Autodesk Fusion 360 part; units mm, degrees
(part 11 of 11)
  spline S89 degree 5 poles (-2.0699, -13.4086) (-2.0698, -13.4117) (-2.0696, -13.4179) (-2.0693, -13.4271) (-2.0688, -13.4395) (-2.0682, -13.4548) (-2.0675, -13.4702) (-2.0667, -13.4855) (-2.0659, -13.5008) (-2.065, -13.516) (-2.064, -13.5312) (-2.063, -13.5464) (-2.0619, -13.5616) (-2.0607, -13.5768) (-2.0595, -13.5919) (-2.0582, -13.6069) (-2.0568, -13.622) (-2.0553, -13.637) (-2.0538, -13.652) (-2.0522, -13.667) (-2.0506, -13.6819) (-2.0488, -13.6968) (-2.047, -13.7116) (-2.0452, -13.7265) (-2.0432, -13.7412) (-2.0412, -13.756) (-2.0391, -13.7707) (-2.0369, -13.7854) (-2.0347, -13.8) (-2.0324, -13.8147) (-2.03, -13.8292) (-2.0275, -13.8438) (-2.025, -13.8583) (-2.0224, -13.8727) (-2.0197, -13.8872) (-2.0169, -13.9015) (-2.0141, -13.9159) (-2.0112, -13.9302) (-2.0082, -13.9444) (-2.0051, -13.9587) (-2.0019, -13.9728) (-1.9987, -13.987) (-1.9954, -14.001) (-1.992, -14.0151) (-1.9885, -14.0291) (-1.9849, -14.043) (-1.9812, -14.0569) (-1.9775, -14.0708) (-1.9737, -14.0846) (-1.9697, -14.0983) (-1.9657, -14.112) (-1.9616, -14.1256) (-1.9574, -14.1392) (-1.9531, -14.1527) (-1.9487, -14.1662) (-1.9442, -14.1796) (-1.9396, -14.193) (-1.9349, -14.2063) (-1.9301, -14.2195) (-1.9252, -14.2327) (-1.9202, -14.2458) (-1.915, -14.2588) (-1.9097, -14.2717) (-1.9042, -14.2845) (-1.8986, -14.2972) (-1.8929, -14.3098) (-1.8871, -14.3224) (-1.8812, -14.335) (-1.8753, -14.3475) (-1.8691, -14.3598) (-1.8626, -14.3719) (-1.857, -14.3814) (-1.8526, -14.3883) (-1.8495, -14.3929) (-1.848, -14.3952) knots -1 -1 -1 -1 -1 -1 -0.98571429 -0.97142857 -0.95714286 -0.94285714 -0.92857143 -0.91428571 -0.9 -0.88571429 -0.87142857 -0.85714286 -0.84285714 -0.82857143 -0.81428571 -0.8 -0.78571429 -0.77142857 -0.75714286 -0.74285714 -0.72857143 -0.71428571 -0.7 -0.68571429 -0.67142857 -0.65714286 -0.64285714 -0.62857143 -0.61428571 -0.6 -0.58571429 -0.57142857 -0.55714286 -0.54285714 -0.52857143 -0.51428571 -0.5 -0.48571429 -0.47142857 -0.45714286 -0.44285714 -0.42857143 -0.41428571 -0.4 -0.38571429 -0.37142857 -0.35714286 -0.34285714 -0.32857143 -0.31428571 -0.3 -0.28571429 -0.27142857 -0.25714286 -0.24285714 -0.22857143 -0.21428571 -0.2 -0.18571429 -0.17142857 -0.15714286 -0.14285714 -0.12857143 -0.11428571 -0.1 -0.08571429 -0.07142857 -0.05714286 -0.04285714 -0.02857143 -0.01428571 0 0 0 0 0 0
  line L97 (-1.848, -14.3952) -> (-1.8092, -14.4516)
  arc A187 (-1.8651, -14.7929) -> (-1.8092, -14.4516) centre (-2.0153, -14.5931) ccw
  arc A188 (-1.8651, -14.7929) -> (-1.9565, -14.8631) centre (1.6741, -19.5) ccw
  arc A189 (-2.3006, -14.8287) -> (-1.9565, -14.8631) centre (-2.1106, -14.6662) ccw
  line L98 (-2.3006, -14.8287) -> (-2.3452, -14.7767)
  spline S90 degree 5 poles (-2.3452, -14.7767) (-2.3469, -14.7746) (-2.3506, -14.7705) (-2.3561, -14.7644) (-2.3639, -14.7566) (-2.3739, -14.7471) (-2.3842, -14.738) (-2.3947, -14.729) (-2.4053, -14.7201) (-2.416, -14.7112) (-2.4267, -14.7024) (-2.4375, -14.6937) (-2.4485, -14.6851) (-2.4596, -14.6766) (-2.4708, -14.6682) (-2.4821, -14.66) (-2.4936, -14.6519) (-2.5051, -14.6438) (-2.5168, -14.6359) (-2.5285, -14.628) (-2.5403, -14.6201) (-2.5521, -14.6124) (-2.5641, -14.6047) (-2.5761, -14.5971) (-2.5882, -14.5896) (-2.6004, -14.5822) (-2.6127, -14.5749) (-2.625, -14.5676) (-2.6374, -14.5604) (-2.6499, -14.5533) (-2.6624, -14.5462) (-2.675, -14.5392) (-2.6877, -14.5323) (-2.7005, -14.5254) (-2.7133, -14.5186) (-2.7261, -14.5119) (-2.7391, -14.5053) (-2.7521, -14.4987) (-2.7651, -14.4922) (-2.7782, -14.4857) (-2.7914, -14.4793) (-2.8047, -14.473) (-2.8179, -14.4667) (-2.8313, -14.4605) (-2.8447, -14.4544) (-2.8582, -14.4483) (-2.8717, -14.4423) (-2.8852, -14.4363) (-2.8989, -14.4304) (-2.9125, -14.4246) (-2.9263, -14.4188) (-2.9401, -14.4131) (-2.9539, -14.4075) (-2.9678, -14.4019) (-2.9817, -14.3964) (-2.9957, -14.3909) (-3.0097, -14.3855) (-3.0238, -14.3802) (-3.0379, -14.3749) (-3.0521, -14.3696) (-3.0663, -14.3645) (-3.0806, -14.3594) (-3.0949, -14.3543) (-3.1093, -14.3493) (-3.1237, -14.3444) (-3.1382, -14.3395) (-3.1527, -14.3347) (-3.1672, -14.3299) (-3.1818, -14.3252) (-3.1965, -14.3206) (-3.2111, -14.316) (-3.2229, -14.3123) (-3.2318, -14.3097) (-3.2377, -14.3079) (-3.2406, -14.307) knots 0 0 0 0 0 0 0.01428571 0.02857143 0.04285714 0.05714286 0.07142857 0.08571429 0.1 0.11428571 0.12857143 0.14285714 0.15714286 0.17142857 0.18571429 0.2 0.21428571 0.22857143 0.24285714 0.25714286 0.27142857 0.28571429 0.3 0.31428571 0.32857143 0.34285714 0.35714286 0.37142857 0.38571429 0.4 0.41428571 0.42857143 0.44285714 0.45714286 0.47142857 0.48571429 0.5 0.51428571 0.52857143 0.54285714 0.55714286 0.57142857 0.58571429 0.6 0.61428571 0.62857143 0.64285714 0.65714286 0.67142857 0.68571429 0.7 0.71428571 0.72857143 0.74285714 0.75714286 0.77142857 0.78571429 0.8 0.81428571 0.82857143 0.84285714 0.85714286 0.87142857 0.88571429 0.9 0.91428571 0.92857143 0.94285714 0.95714286 0.97142857 0.98571429 1 1 1 1 1 1
  arc A190 (-3.2406, -14.307) -> (-3.5189, -14.5852) centre (1.6741, -19.5) ccw
  spline S91 degree 5 poles (-3.5189, -14.5852) (-3.518, -14.5882) (-3.5162, -14.5941) (-3.5135, -14.6029) (-3.5099, -14.6147) (-3.5053, -14.6294) (-3.5007, -14.644) (-3.496, -14.6586) (-3.4912, -14.6732) (-3.4864, -14.6877) (-3.4815, -14.7021) (-3.4766, -14.7166) (-3.4716, -14.7309) (-3.4665, -14.7452) (-3.4614, -14.7595) (-3.4562, -14.7737) (-3.451, -14.7879) (-3.4457, -14.8021) (-3.4404, -14.8161) (-3.435, -14.8302) (-3.4295, -14.8442) (-3.424, -14.8581) (-3.4184, -14.872) (-3.4127, -14.8858) (-3.407, -14.8996) (-3.4012, -14.9133) (-3.3954, -14.927) (-3.3895, -14.9406) (-3.3836, -14.9542) (-3.3776, -14.9677) (-3.3715, -14.9812) (-3.3653, -14.9946) (-3.3591, -15.0079) (-3.3529, -15.0212) (-3.3466, -15.0344) (-3.3402, -15.0476) (-3.3337, -15.0607) (-3.3272, -15.0738) (-3.3206, -15.0868) (-3.3139, -15.0997) (-3.3072, -15.1126) (-3.3004, -15.1254) (-3.2936, -15.1382) (-3.2866, -15.1508) (-3.2797, -15.1634) (-3.2726, -15.176) (-3.2655, -15.1885) (-3.2583, -15.2009) (-3.251, -15.2132) (-3.2436, -15.2255) (-3.2362, -15.2377) (-3.2287, -15.2498) (-3.2211, -15.2618) (-3.2135, -15.2737) (-3.2057, -15.2856) (-3.1979, -15.2974) (-3.19, -15.3091) (-3.182, -15.3207) (-3.174, -15.3323) (-3.1659, -15.3437) (-3.1576, -15.3551) (-3.1493, -15.3663) (-3.1408, -15.3774) (-3.1322, -15.3883) (-3.1235, -15.3992) (-3.1147, -15.4099) (-3.1058, -15.4206) (-3.0969, -15.4312) (-3.0879, -15.4417) (-3.0787, -15.452) (-3.0693, -15.462) (-3.0615, -15.4697) (-3.0554, -15.4753) (-3.0513, -15.4789) (-3.0492, -15.4807) knots -1 -1 -1 -1 -1 -1 -0.98571429 -0.97142857 -0.95714286 -0.94285714 -0.92857143 -0.91428571 -0.9 -0.88571429 -0.87142857 -0.85714286 -0.84285714 -0.82857143 -0.81428571 -0.8 -0.78571429 -0.77142857 -0.75714286 -0.74285714 -0.72857143 -0.71428571 -0.7 -0.68571429 -0.67142857 -0.65714286 -0.64285714 -0.62857143 -0.61428571 -0.6 -0.58571429 -0.57142857 -0.55714286 -0.54285714 -0.52857143 -0.51428571 -0.5 -0.48571429 -0.47142857 -0.45714286 -0.44285714 -0.42857143 -0.41428571 -0.4 -0.38571429 -0.37142857 -0.35714286 -0.34285714 -0.32857143 -0.31428571 -0.3 -0.28571429 -0.27142857 -0.25714286 -0.24285714 -0.22857143 -0.21428571 -0.2 -0.18571429 -0.17142857 -0.15714286 -0.14285714 -0.12857143 -0.11428571 -0.1 -0.08571429 -0.07142857 -0.05714286 -0.04285714 -0.02857143 -0.01428571 0 0 0 0 0 0
  line L99 (-3.0492, -15.4807) -> (-2.9971, -15.5252)
  arc A191 (-2.9628, -15.8693) -> (-2.9971, -15.5252) centre (-3.1596, -15.7152) ccw
  arc A192 (-2.9628, -15.8693) -> (-3.0329, -15.9608) centre (1.6741, -19.5) ccw
  arc A193 (-3.3742, -16.0167) -> (-3.0329, -15.9608) centre (-3.2328, -15.8105) ccw
  line L100 (-3.3742, -16.0167) -> (-3.4307, -15.9779)
  spline S92 degree 5 poles (-3.4307, -15.9779) (-3.433, -15.9763) (-3.4375, -15.9733) (-3.4445, -15.9689) (-3.454, -15.9633) (-3.4661, -15.9568) (-3.4784, -15.9506) (-3.4909, -15.9446) (-3.5034, -15.9388) (-3.516, -15.933) (-3.5287, -15.9272) (-3.5414, -15.9216) (-3.5542, -15.9162) (-3.5671, -15.9108) (-3.5801, -15.9057) (-3.5932, -15.9006) (-3.6064, -15.8957) (-3.6196, -15.891) (-3.6329, -15.8863) (-3.6463, -15.8817) (-3.6597, -15.8772) (-3.6731, -15.8728) (-3.6866, -15.8685) (-3.7002, -15.8642) (-3.7139, -15.8601) (-3.7276, -15.8561) (-3.7413, -15.8522) (-3.7551, -15.8484) (-3.769, -15.8446) (-3.7829, -15.841) (-3.7968, -15.8374) (-3.8108, -15.8339) (-3.8248, -15.8305) (-3.8389, -15.8272) (-3.853, -15.8239) (-3.8672, -15.8208) (-3.8814, -15.8177) (-3.8957, -15.8147) (-3.91, -15.8118) (-3.9243, -15.8089) (-3.9387, -15.8062) (-3.9531, -15.8035) (-3.9676, -15.8009) (-3.9821, -15.7983) (-3.9966, -15.7959) (-4.0112, -15.7935) (-4.0258, -15.7912) (-4.0405, -15.7889) (-4.0551, -15.7868) (-4.0699, -15.7847) (-4.0846, -15.7827) (-4.0994, -15.7807) (-4.1142, -15.7788) (-4.1291, -15.777) (-4.144, -15.7753) (-4.1589, -15.7736) (-4.1739, -15.772) (-4.1888, -15.7705) (-4.2039, -15.7691) (-4.2189, -15.7677) (-4.234, -15.7664) (-4.2491, -15.7651) (-4.2642, -15.764) (-4.2794, -15.7629) (-4.2946, -15.7618) (-4.3098, -15.7609) (-4.3251, -15.76) (-4.3404, -15.7591) (-4.3557, -15.7583) (-4.371, -15.7576) (-4.3864, -15.757) (-4.3987, -15.7566) (-4.408, -15.7562) (-4.4141, -15.7561) (-4.4172, -15.756) knots 0 0 0 0 0 0 0.01428571 0.02857143 0.04285714 0.05714286 0.07142857 0.08571429 0.1 0.11428571 0.12857143 0.14285714 0.15714286 0.17142857 0.18571429 0.2 0.21428571 0.22857143 0.24285714 0.25714286 0.27142857 0.28571429 0.3 0.31428571 0.32857143 0.34285714 0.35714286 0.37142857 0.38571429 0.4 0.41428571 0.42857143 0.44285714 0.45714286 0.47142857 0.48571429 0.5 0.51428571 0.52857143 0.54285714 0.55714286 0.57142857 0.58571429 0.6 0.61428571 0.62857143 0.64285714 0.65714286 0.67142857 0.68571429 0.7 0.71428571 0.72857143 0.74285714 0.75714286 0.77142857 0.78571429 0.8 0.81428571 0.82857143 0.84285714 0.85714286 0.87142857 0.88571429 0.9 0.91428571 0.92857143 0.94285714 0.95714286 0.97142857 0.98571429 1 1 1 1 1 1
  arc A194 (-4.4172, -15.756) -> (-4.614, -16.0967) centre (1.6741, -19.5) ccw
  spline S93 degree 5 poles (-4.614, -16.0967) (-4.6123, -16.0994) (-4.6091, -16.1046) (-4.6042, -16.1125) (-4.5977, -16.1229) (-4.5894, -16.1359) (-4.5811, -16.1488) (-4.5728, -16.1617) (-4.5645, -16.1745) (-4.556, -16.1873) (-4.5476, -16.2) (-4.5391, -16.2126) (-4.5306, -16.2252) (-4.522, -16.2378) (-4.5133, -16.2502) (-4.5047, -16.2626) (-4.4959, -16.275) (-4.4872, -16.2872) (-4.4784, -16.2995) (-4.4695, -16.3116) (-4.4606, -16.3237) (-4.4517, -16.3357) (-4.4427, -16.3477) (-4.4336, -16.3596) (-4.4246, -16.3714) (-4.4154, -16.3832) (-4.4063, -16.3949) (-4.397, -16.4065) (-4.3878, -16.4181) (-4.3785, -16.4296) (-4.3691, -16.441) (-4.3597, -16.4524) (-4.3503, -16.4637) (-4.3408, -16.4749) (-4.3312, -16.4861) (-4.3217, -16.4971) (-4.312, -16.5081) (-4.3023, -16.5191) (-4.2926, -16.5299) (-4.2828, -16.5407) (-4.273, -16.5514) (-4.2632, -16.562) (-4.2532, -16.5725) (-4.2433, -16.583) (-4.2332, -16.5933) (-4.2232, -16.6036) (-4.2131, -16.6138) (-4.2029, -16.624) (-4.1927, -16.634) (-4.1824, -16.6439) (-4.1721, -16.6538) (-4.1617, -16.6635) (-4.1513, -16.6732) (-4.1408, -16.6827) (-4.1302, -16.6922) (-4.1196, -16.7016) (-4.109, -16.7108) (-4.0982, -16.72) (-4.0875, -16.7291) (-4.0767, -16.738) (-4.0658, -16.7469) (-4.0548, -16.7555) (-4.0437, -16.764) (-4.0326, -16.7724) (-4.0214, -16.7806) (-4.0101, -16.7887) (-3.9988, -16.7967) (-3.9874, -16.8047) (-3.976, -16.8125) (-3.9645, -16.82) (-3.9528, -16.8273) (-3.9432, -16.8327) (-3.9359, -16.8365) (-3.931, -16.839) (-3.9285, -16.8401) knots -1 -1 -1 -1 -1 -1 -0.98571429 -0.97142857 -0.95714286 -0.94285714 -0.92857143 -0.91428571 -0.9 -0.88571429 -0.87142857 -0.85714286 -0.84285714 -0.82857143 -0.81428571 -0.8 -0.78571429 -0.77142857 -0.75714286 -0.74285714 -0.72857143 -0.71428571 -0.7 -0.68571429 -0.67142857 -0.65714286 -0.64285714 -0.62857143 -0.61428571 -0.6 -0.58571429 -0.57142857 -0.55714286 -0.54285714 -0.52857143 -0.51428571 -0.5 -0.48571429 -0.47142857 -0.45714286 -0.44285714 -0.42857143 -0.41428571 -0.4 -0.38571429 -0.37142857 -0.35714286 -0.34285714 -0.32857143 -0.31428571 -0.3 -0.28571429 -0.27142857 -0.25714286 -0.24285714 -0.22857143 -0.21428571 -0.2 -0.18571429 -0.17142857 -0.15714286 -0.14285714 -0.12857143 -0.11428571 -0.1 -0.08571429 -0.07142857 -0.05714286 -0.04285714 -0.02857143 -0.01428571 0 0 0 0 0 0
  line L101 (-3.9285, -16.8401) -> (-3.8667, -16.8697)
  arc A195 (-3.7445, -17.1932) -> (-3.8667, -16.8697) centre (-3.9745, -17.0952) ccw
  arc A196 (-3.7445, -17.1932) -> (-3.7886, -17.2996) centre (1.6741, -19.5) ccw
  arc A197 (-4.1038, -17.442) -> (-3.7886, -17.2996) centre (-4.0205, -17.2062) ccw
  line L102 (-4.1038, -17.442) -> (-4.1683, -17.4191)
  spline S94 degree 5 poles (-4.1683, -17.4191) (-4.1709, -17.4182) (-4.1761, -17.4165) (-4.184, -17.414) (-4.1946, -17.4111) (-4.208, -17.4079) (-4.2215, -17.4051) (-4.2351, -17.4026) (-4.2487, -17.4002) (-4.2624, -17.3978) (-4.2761, -17.3956) (-4.2898, -17.3934) (-4.3036, -17.3915) (-4.3175, -17.3897) (-4.3314, -17.388) (-4.3453, -17.3866) (-4.3593, -17.3853) (-4.3733, -17.3841) (-4.3874, -17.383) (-4.4015, -17.382) (-4.4156, -17.3811) (-4.4297, -17.3803) (-4.4439, -17.3797) (-4.4581, -17.3791) (-4.4723, -17.3787) (-4.4866, -17.3783) (-4.5009, -17.3781) (-4.5152, -17.378) (-4.5296, -17.378) (-4.5439, -17.378) (-4.5583, -17.3782) (-4.5728, -17.3784) (-4.5872, -17.3788) (-4.6017, -17.3792) (-4.6161, -17.3797) (-4.6306, -17.3803) (-4.6452, -17.381) (-4.6597, -17.3818) (-4.6743, -17.3827) (-4.6889, -17.3837) (-4.7035, -17.3847) (-4.7181, -17.3859) (-4.7328, -17.3871) (-4.7474, -17.3884) (-4.7621, -17.3898) (-4.7768, -17.3912) (-4.7915, -17.3928) (-4.8062, -17.3944) (-4.821, -17.3961) (-4.8357, -17.3979) (-4.8505, -17.3998) (-4.8653, -17.4017) (-4.8801, -17.4038) (-4.8949, -17.4059) (-4.9098, -17.4081) (-4.9246, -17.4103) (-4.9395, -17.4126) (-4.9543, -17.4151) (-4.9692, -17.4175) (-4.9841, -17.4201) (-4.999, -17.4227) (-5.0139, -17.4255) (-5.0289, -17.4282) (-5.0438, -17.4311) (-5.0587, -17.434) (-5.0737, -17.437) (-5.0887, -17.4401) (-5.1037, -17.4433) (-5.1186, -17.4465) (-5.1336, -17.4498) (-5.1486, -17.4531) (-5.1607, -17.4559) (-5.1697, -17.458) (-5.1757, -17.4594) (-5.1787, -17.4601) knots 0 0 0 0 0 0 0.01428571 0.02857143 0.04285714 0.05714286 0.07142857 0.08571429 0.1 0.11428571 0.12857143 0.14285714 0.15714286 0.17142857 0.18571429 0.2 0.21428571 0.22857143 0.24285714 0.25714286 0.27142857 0.28571429 0.3 0.31428571 0.32857143 0.34285714 0.35714286 0.37142857 0.38571429 0.4 0.41428571 0.42857143 0.44285714 0.45714286 0.47142857 0.48571429 0.5 0.51428571 0.52857143 0.54285714 0.55714286 0.57142857 0.58571429 0.6 0.61428571 0.62857143 0.64285714 0.65714286 0.67142857 0.68571429 0.7 0.71428571 0.72857143 0.74285714 0.75714286 0.77142857 0.78571429 0.8 0.81428571 0.82857143 0.84285714 0.85714286 0.87142857 0.88571429 0.9 0.91428571 0.92857143 0.94285714 0.95714286 0.97142857 0.98571429 1 1 1 1 1 1
  arc A198 (-5.1787, -17.4601) -> (-5.2805, -17.8402) centre (1.6741, -19.5) ccw
  spline S95 degree 5 poles (-5.2805, -17.8402) (-5.2783, -17.8423) (-5.2738, -17.8465) (-5.267, -17.8529) (-5.258, -17.8612) (-5.2467, -17.8717) (-5.2353, -17.882) (-5.224, -17.8923) (-5.2126, -17.9025) (-5.2012, -17.9127) (-5.1897, -17.9227) (-5.1782, -17.9328) (-5.1667, -17.9427) (-5.1552, -17.9526) (-5.1436, -17.9624) (-5.132, -17.9721) (-5.1204, -17.9818) (-5.1088, -17.9914) (-5.0971, -18.0009) (-5.0854, -18.0104) (-5.0737, -18.0197) (-5.0619, -18.029) (-5.0501, -18.0383) (-5.0383, -18.0474) (-5.0265, -18.0565) (-5.0146, -18.0655) (-5.0027, -18.0744) (-4.9908, -18.0833) (-4.9789, -18.0921) (-4.9669, -18.1008) (-4.9549, -18.1094) (-4.9429, -18.1179) (-4.9309, -18.1264) (-4.9188, -18.1348) (-4.9067, -18.1431) (-4.8946, -18.1513) (-4.8824, -18.1594) (-4.8702, -18.1675) (-4.858, -18.1754) (-4.8458, -18.1833) (-4.8335, -18.1911) (-4.8213, -18.1988) (-4.809, -18.2064) (-4.7966, -18.2139) (-4.7843, -18.2213) (-4.7719, -18.2287) (-4.7595, -18.2359) (-4.747, -18.243) (-4.7345, -18.2501) (-4.722, -18.257) (-4.7095, -18.2639) (-4.697, -18.2706) (-4.6844, -18.2772) (-4.6718, -18.2838) (-4.6591, -18.2901) (-4.6465, -18.2964) (-4.6338, -18.3026) (-4.6211, -18.3087) (-4.6083, -18.3147) (-4.5956, -18.3206) (-4.5828, -18.3263) (-4.5699, -18.3318) (-4.557, -18.3372) (-4.5441, -18.3423) (-4.5311, -18.3474) (-4.5181, -18.3523) (-4.5051, -18.3571) (-4.4921, -18.3618) (-4.4791, -18.3664) (-4.466, -18.3707) (-4.4528, -18.3747) (-4.4422, -18.3775) (-4.4341, -18.3793) (-4.4287, -18.3803) (-4.426, -18.3808) knots -1 -1 -1 -1 -1 -1 -0.98571429 -0.97142857 -0.95714286 -0.94285714 -0.92857143 -0.91428571 -0.9 -0.88571429 -0.87142857 -0.85714286 -0.84285714 -0.82857143 -0.81428571 -0.8 -0.78571429 -0.77142857 -0.75714286 -0.74285714 -0.72857143 -0.71428571 -0.7 -0.68571429 -0.67142857 -0.65714286 -0.64285714 -0.62857143 -0.61428571 -0.6 -0.58571429 -0.57142857 -0.55714286 -0.54285714 -0.52857143 -0.51428571 -0.5 -0.48571429 -0.47142857 -0.45714286 -0.44285714 -0.42857143 -0.41428571 -0.4 -0.38571429 -0.37142857 -0.35714286 -0.34285714 -0.32857143 -0.31428571 -0.3 -0.28571429 -0.27142857 -0.25714286 -0.24285714 -0.22857143 -0.21428571 -0.2 -0.18571429 -0.17142857 -0.15714286 -0.14285714 -0.12857143 -0.11428571 -0.1 -0.08571429 -0.07142857 -0.05714286 -0.04285714 -0.02857143 -0.01428571 0 0 0 0 0 0
  line L103 (-4.426, -18.3808) -> (-4.3587, -18.3934)
  arc A199 (-4.1569, -18.6742) -> (-4.3587, -18.3934) centre (-4.4044, -18.6392) ccw
  circle A200 centre (1.6741, -19.5) radius 1.25
  line L104 (-5, -26) -> (-5, -5)
  circle A201 centre (3, -17) radius 0.9
  dimension "d200" = 1.8
  constraint midpoint L51 L104.start
  constraint midpoint L55 L104.end
  constraint symmetric A97 L104 A201
  measures "d200" diameter of A97
extrude "Extrude3" add sketch "Sketch22" along normal blind 1.5 separate body contours A97 sketch seen with x (1, 0, 0) y (0, 1, 0) z (0, 0, 1) at (-11.6741, -19.5, -3.25) makes body 5 in component "Spur Gear (24 teeth)"
hole "Hole1" at (15.3685, 17.4789, 5.45) direction (0, 0, 1) diameter 1.9 depth 1.5 tip angle 118 bodies 4 in component "Component"
extrude "Extrude3'" add sketch "Sketch22" along normal blind 1.5 contours A201 sketch seen with x (1, 0, 0) y (0, 1, 0) z (0, 0, 1) at (1.6741, -19.5, -3.25) bodies 3 in component "Spur Gear (24 teeth) (1)"
copy_body "Body->Comp11" bodies 1 removing the originals makes body 6 in component "Component'"
sketch "Sketch23" plane through (0, 0, 8.2) normal (0, 0, 1) x (-1, 0, 0)
  circle A0 centre (-12.6464, -16.8424) radius 0.1179
  line L0 (-21.5245, -12.7207) -> (-11.2176, -18.8662)
  line L1 (-11.2176, -18.8662) -> (-10.1934, -17.1484)
  line L2 (-10.1934, -17.1484) -> (-20.5003, -11.0028)
  line L3 (-20.5003, -11.0028) -> (-21.5245, -12.7207)
  circle A1 centre (-19.4042, -12.827) radius 0.9
  line L4 (-5, -23) -> (-5, -2)
  circle A2 centre (13, -13) radius 0.9
  dimension "d221" = 1.8
  dimension "d222" = 1.8
  constraint vertical L4
  measures "d221" diameter of A1
  measures "d222" diameter of A2
extrude "Extrude2''" add sketch "Sketch23" along normal blind 10 contours A1 sketch seen with x (0.990644, 0.136473, 0) y (-0.136473, 0.990644, 0) z (0, 0, 1) at (5.1389, -0.9319, -0.75) bodies 4 in component "Component"
sketch "Sketch25" plane through (0, 0, 0) normal (0, 0, 1) x (1, 0, 0)
  line L0 (0, 0) -> (10, 0)
  line L1 (10, 0) -> (10, 2)
  line L2 (10, 2) -> (0, 2)
  line L3 (0, 2) -> (0, 0)
  dimension "d246" = 10
  constraint horizontal L0
  constraint vertical L1
  constraint horizontal L2
  constraint vertical L3
  constraint coincident L0.start L3.end
  measures "d246" distance of L0.start L0.end
extrude "Extrude18" add sketch "Sketch25" along normal blind 2 separate body makes body 7
copy_body "Body->Comp12" bodies 7 removing the originals makes body 8 in component "Component''"
sketch "Sketch26" plane through (0, 0, 0) normal (0, 0, -1) x (1, 0, 0)
  line L0 (0, 0) -> (0, -2)
  line L1 (0, -2) -> (10, -2)
  line L2 (10, -2) -> (10, 0)
  line L3 (10, 0) -> (0, 0)
  line L4 (-13, 0) -> (-13, -2)
  line L5 (-13, -2) -> (-3, -2)
  line L6 (-3, -2) -> (-3, 0)
  line L7 (-3, 0) -> (-13, 0)
  circle A0 centre (7.5, -1) radius 0.9
  circle A1 centre (-5.5, -0.9885) radius 0.9
  dimension "d234" = 1.8
  dimension "d235" = 1.8
  dimension "d247" = 2.5
  dimension "d248" = 2.5
  measures "d234" diameter of A0
  measures "d235" diameter of A1
  measures "d247" distance of L6 A1.centre
  measures "d248" distance of L2 A0.centre
extrude "Extrude1'''" cut sketch "Sketch26" against normal blind 4 contours A0 | A1 bodies 8 in component "Component''"
sketch "Sketch29" plane through (0, 0, 0) normal (0, 0, 1) x (1, 0, 0)
  line L0 (0, 0) -> (10, 0)
  line L1 (10, 0) -> (10, 2)
  line L2 (10, 2) -> (0, 2)
  line L3 (0, 2) -> (0, 0)
  dimension "d255" = 10
  dimension "d256" = 2
  constraint horizontal L0
  constraint vertical L1
  constraint horizontal L2
  constraint vertical L3
  constraint coincident L0.start L3.end
  measures "d255" distance of L0.start L0.end
  measures "d256" distance of L0.start L2.end
extrude "Extrude20" add sketch "Sketch29" along normal blind 2 separate body makes body 9
copy_body "CopyPasteBodies1" bodies 9 makes body 10
move_body "Move1" bodies 10 to x (1, 0, 0) y (0, 1, 0) z (0, 0, 1) at (-11.5, 0, 0)
copy_body "Body->Comp14" bodies 9 removing the originals makes body 11 in component "Component'''"
copy_body "Body->Comp15" bodies 10 removing the originals makes body 12 in component "Component''''"
sketch "Sketch30" plane through (0, 0, 2) normal (0, 0, 1) x (-1, 0, 0)
  line L0 (0, -2) -> (0, 0)
  line L1 (0, 0) -> (-10, 0)
  line L2 (-10, 0) -> (-10, -2)
  line L3 (-10, -2) -> (0, -2)
  circle A0 centre (-1.5, -1) radius 0.9
  circle A1 centre (3, -1) radius 0.9
  dimension "d259" = 1.8
  dimension "d261" = 1.8
  measures "d259" diameter of A0
  measures "d261" diameter of A1
extrude "Extrude1''''" cut sketch "Sketch30" against normal blind 3.5 contours A0 | A1 bodies 11 in component "Component'''"
extrude "Extrude1'''''" cut sketch "Sketch30" against normal blind 3.5 contours A0 | A1 bodies 12 in component "Component''''"
sketch "Sketch31" plane through (0, 0, 0) normal (0, 0, 1) x (1, 0, 0)
  line L0 (45, 0) -> (50, 0)
  line L1 (45, 0) -> (45, 10)
  line L2 (45, 10) -> (45, 10.3239)
  line L3 (45, 10.3239) -> (50, 15)
  line L4 (50, 15) -> (50, 11)
  line L5 (50, 11) -> (49, 11)
  arc A0 (49, 11) -> (49, 10) centre (49, 10.5) ccw
  line L6 (49, 10) -> (50, 10)
  line L7 (50, 10) -> (50, 0)
  line L8 (53, 15) -> (53, 0)
  line L9 (56, 10) -> (56, 0)
  line L10 (61, 10) -> (61, 10.3239)
  line L11 (61, 10.3239) -> (56, 15)
  arc A1 (57, 10) -> (57, 11) centre (57, 10.5) ccw
  line L12 (61, 0) -> (56, 0)
  line L13 (56, 11) -> (57, 11)
  line L14 (57, 10) -> (56, 10)
  line L15 (61, 0) -> (61, 10)
  line L16 (56, 15) -> (56, 11)
  constraint horizontal L0
  constraint perpendicular L0 L1
  constraint perpendicular L0 L2
  constraint parallel L2 L4
  constraint perpendicular L4 L5
  constraint tangent L5 A0
  constraint tangent A0 L6
  constraint perpendicular L4 L6
  constraint perpendicular L0 L7
  constraint vertical L8
  constraint symmetric L0.start L8 L12.start
  constraint symmetric L0.end L8 L9.end
  constraint symmetric L1.end L8 L10.start
  constraint symmetric L2.end L8 L10.end
  constraint symmetric L3.end L8 L11.end
  constraint symmetric L4.end L8 L13.start
  constraint symmetric L5.end L8 A1.end
  constraint symmetric A0.end L8 A1.start
  constraint symmetric A0 L8 A1
  constraint symmetric L6.end L8 L9.start
extrude "Extrude1''''''" add sketch "Sketch31" along normal blind 4.1 separate body contours L0 L1 L2 L3 L4 L5 A0 L6 L7 makes body 13 in component "Component'''''"
extrude "Extrude1'''''''" add sketch "Sketch31" along normal blind 4.1 separate body contours L9 L10 L11 A1 L12 L13 L14 L15 L16 makes body 14 in component "Component''''''"
component "Spur Gear (24 teeth)" placed x (0.990644, -0.136473, 0) y (0.136473, 0.990644, 0) z (0, 0, 1) at (16.8644, 9.8447, 4.8835)
component "Spur Gear (24 teeth) (1)" placed x (1, 0, 0) y (0, 1, 0) z (0, 0, 1) at (3.5161, 9.8447, 4.8835)
component "Component" placed x (0.990644, -0.136473, 0) y (0.136473, 0.990644, 0) z (0, 0, 1) at (0.2266, -8.0309, 2.3835)
component "Component'" placed x (1, 0, 0) y (0, 1, 0) z (0, 0, 1) at (5.1903, -9.6553, 1.6335)
component "Component" placed x (-0.642788, -0.766044, 0) y (0.766044, -0.642788, 0) z (0, 0, 1) at (-1.3207, 30.3528, 2.3835)
component "Component''" placed x (-0.858568, 0.5127, 0) y (-0.5127, -0.858568, 0) z (0, 0, 1) at (31.5465, 0.185, 10.8335)
component "Component''" placed x (0.882948, 0.469472, 0) y (-0.469472, 0.882948, 0) z (0, 0, 1) at (-10.9585, -0.6434, 10.8335)
component "Component'''" placed x (0.858568, -0.5127, 0) y (0.5127, 0.858568, 0) z (0, 0, 1) at (22.794, 3.0822, 16.8335)
component "Component''''" placed x (0.882948, 0.469472, 0) y (-0.469472, 0.882948, 0) z (0, 0, 1) at (-1.6876, 4.2861, 16.8335)
component "Component'''''" placed x (-0.469472, 0.882948, 0) y (-0.882948, -0.469472, 0) z (0, 0, 1) at (15.0519, -38.9116, 12.8335)
component "Component''''''" placed x (-0.497638, -0.867385, 0) y (0.867385, -0.497638, 0) z (0, 0, 1) at (56.4926, 51.668, 12.8335)
